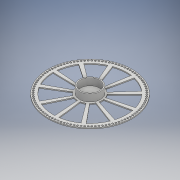
# Autodesk Inventor part: WheeledGrabber
Saved by Autodesk Inventor 2017 (Build 210142000, 142)
## iProperties
Created: 2017-01-07
Part Number: WheeledGrabber
Material: Generic
Document SubType Name: Modeling
Designer: kurti
Density: 1 g/cm^3
Appearance: Default
Author: kurti
Autodesk Inventor part; units mm, degrees
ref_plane "YZ Plane" through (0, 0, 0) normal (1, 0, 0) x (0, 1, 0)
ref_plane "XZ Plane" through (0, 0, 0) normal (0, 1, 0) x (-1, 0, 0)
ref_plane "XY Plane" through (0, 0, 0) normal (0, 0, 1) x (1, 0, 0)
sketch "Sketch1" plane through (0, 0, 0) normal (0, 0, 1) x (1, 0, 0)
  circle A0 centre (0, 0) radius 120
  line L0 (0, 0) -> (0, 115) construction
  circle A1 centre (0, 115) radius 2.5
  circle A2 centre (-7.2209, 114.7731) radius 2.5
  circle A3 centre (-14.4133, 114.0932) radius 2.5
  circle A4 centre (-21.5489, 112.963) radius 2.5
  circle A5 centre (-28.5993, 111.3871) radius 2.5
  circle A6 centre (-35.537, 109.3715) radius 2.5
  circle A7 centre (-42.3343, 106.9243) radius 2.5
  circle A8 centre (-48.9646, 104.0551) radius 2.5
  circle A9 centre (-55.4017, 100.7753) radius 2.5
  circle A10 centre (-61.6201, 97.0977) radius 2.5
  circle A11 centre (-67.5953, 93.037) radius 2.5
  circle A12 centre (-73.3038, 88.609) radius 2.5
  circle A13 centre (-78.7229, 83.8314) radius 2.5
  circle A14 centre (-83.8314, 78.7229) radius 2.5
  circle A15 centre (-88.609, 73.3038) radius 2.5
  circle A16 centre (-93.037, 67.5953) radius 2.5
  circle A17 centre (-97.0977, 61.6201) radius 2.5
  circle A18 centre (-100.7753, 55.4017) radius 2.5
  circle A19 centre (-104.0551, 48.9646) radius 2.5
  circle A20 centre (-106.9243, 42.3343) radius 2.5
  circle A21 centre (-109.3715, 35.537) radius 2.5
  circle A22 centre (-111.3871, 28.5993) radius 2.5
  circle A23 centre (-112.963, 21.5489) radius 2.5
  circle A24 centre (-114.0932, 14.4133) radius 2.5
  circle A25 centre (-114.7731, 7.2209) radius 2.5
  circle A26 centre (-115, 0) radius 2.5
  circle A27 centre (-114.7731, -7.2209) radius 2.5
  circle A28 centre (-114.0932, -14.4133) radius 2.5
  circle A29 centre (-112.963, -21.5489) radius 2.5
  circle A30 centre (-111.3871, -28.5993) radius 2.5
  circle A31 centre (-109.3715, -35.537) radius 2.5
  circle A32 centre (-106.9243, -42.3343) radius 2.5
  circle A33 centre (-104.0551, -48.9646) radius 2.5
  circle A34 centre (-100.7753, -55.4017) radius 2.5
  circle A35 centre (-97.0977, -61.6201) radius 2.5
  circle A36 centre (-93.037, -67.5953) radius 2.5
  circle A37 centre (-88.609, -73.3038) radius 2.5
  circle A38 centre (-83.8314, -78.7229) radius 2.5
  circle A39 centre (-78.7229, -83.8314) radius 2.5
  circle A40 centre (-73.3038, -88.609) radius 2.5
  circle A41 centre (-67.5953, -93.037) radius 2.5
  circle A42 centre (-61.6201, -97.0977) radius 2.5
  circle A43 centre (-55.4017, -100.7753) radius 2.5
  circle A44 centre (-48.9646, -104.0551) radius 2.5
  circle A45 centre (-42.3343, -106.9243) radius 2.5
  circle A46 centre (-35.537, -109.3715) radius 2.5
  circle A47 centre (-28.5993, -111.3871) radius 2.5
  circle A48 centre (-21.5489, -112.963) radius 2.5
  circle A49 centre (-14.4133, -114.0932) radius 2.5
  circle A50 centre (-7.2209, -114.7731) radius 2.5
  circle A51 centre (0, -115) radius 2.5
  circle A52 centre (7.2209, -114.7731) radius 2.5
  circle A53 centre (14.4133, -114.0932) radius 2.5
  circle A54 centre (21.5489, -112.963) radius 2.5
  circle A55 centre (28.5993, -111.3871) radius 2.5
  circle A56 centre (35.537, -109.3715) radius 2.5
  circle A57 centre (42.3343, -106.9243) radius 2.5
  circle A58 centre (48.9646, -104.0551) radius 2.5
  circle A59 centre (55.4017, -100.7753) radius 2.5
  circle A60 centre (61.6201, -97.0977) radius 2.5
  circle A61 centre (67.5953, -93.037) radius 2.5
  circle A62 centre (73.3038, -88.609) radius 2.5
  circle A63 centre (78.7229, -83.8314) radius 2.5
  circle A64 centre (83.8314, -78.7229) radius 2.5
  circle A65 centre (88.609, -73.3038) radius 2.5
  circle A66 centre (93.037, -67.5953) radius 2.5
  circle A67 centre (97.0977, -61.6201) radius 2.5
  circle A68 centre (100.7753, -55.4017) radius 2.5
  circle A69 centre (104.0551, -48.9646) radius 2.5
  circle A70 centre (106.9243, -42.3343) radius 2.5
  circle A71 centre (109.3715, -35.537) radius 2.5
  circle A72 centre (111.3871, -28.5993) radius 2.5
  circle A73 centre (112.963, -21.5489) radius 2.5
  circle A74 centre (114.0932, -14.4133) radius 2.5
  circle A75 centre (114.7731, -7.2209) radius 2.5
  circle A76 centre (115, 0) radius 2.5
  circle A77 centre (114.7731, 7.2209) radius 2.5
  circle A78 centre (114.0932, 14.4133) radius 2.5
  circle A79 centre (112.963, 21.5489) radius 2.5
  circle A80 centre (111.3871, 28.5993) radius 2.5
  circle A81 centre (109.3715, 35.537) radius 2.5
  circle A82 centre (106.9243, 42.3343) radius 2.5
  circle A83 centre (104.0551, 48.9646) radius 2.5
  circle A84 centre (100.7753, 55.4017) radius 2.5
  circle A85 centre (97.0977, 61.6201) radius 2.5
  circle A86 centre (93.037, 67.5953) radius 2.5
  circle A87 centre (88.609, 73.3038) radius 2.5
  circle A88 centre (83.8314, 78.7229) radius 2.5
  circle A89 centre (78.7229, 83.8314) radius 2.5
  circle A90 centre (73.3038, 88.609) radius 2.5
  circle A91 centre (67.5953, 93.037) radius 2.5
  circle A92 centre (61.6201, 97.0977) radius 2.5
  circle A93 centre (55.4017, 100.7753) radius 2.5
  circle A94 centre (48.9646, 104.0551) radius 2.5
  circle A95 centre (42.3343, 106.9243) radius 2.5
  circle A96 centre (35.537, 109.3715) radius 2.5
  circle A97 centre (28.5993, 111.3871) radius 2.5
  circle A98 centre (21.5489, 112.963) radius 2.5
  circle A99 centre (14.4133, 114.0932) radius 2.5
  circle A100 centre (7.2209, 114.7731) radius 2.5
  line L1 (0, 0) -> (90.9327, 52.5) construction
  line L2 (0, 0) -> (105, 0) construction
  line L3 (90.9327, 52.5) -> (8.6603, 5) construction
  line L4 (8.6603, 5) -> (75.8354, 72.1751)
  line L5 (8.6603, 5) -> (100.4232, 29.5878)
  line L6 (8.6603, 5) -> (103.6603, 5) construction
  arc A101 (100.4232, 29.5878) -> (75.8354, 72.1751) centre (-0.2751, -0.1588) ccw
  line L7 (4.4527, 9.0118) -> (24.6465, 101.8408)
  arc A102 (68.3555, 79.3072) -> (24.6465, 101.8408) centre (-0.2751, -0.1588) ccw
  line L8 (4.4527, 9.0118) -> (68.3555, 79.3072)
  line L9 (-1.2558, 10.1121) -> (-34.4549, 99.1223)
  arc A103 (14.498, 103.7967) -> (-34.4549, 99.1223) centre (-0.2751, -0.1588) ccw
  line L10 (-1.2558, 10.1121) -> (14.498, 103.7967)
  line L11 (-6.653, 7.9514) -> (-82.7044, 64.8828)
  arc A104 (-44.0497, 95.2811) -> (-82.7044, 64.8828) centre (-0.2751, -0.1588) ccw
  line L12 (-6.653, 7.9514) -> (-44.0497, 95.2811)
  line L13 (-10.0252, 3.2158) -> (-104.7831, 9.993)
  arc A105 (-88.6994, 56.464) -> (-104.7831, 9.993) centre (-0.2751, -0.1588) ccw
  line L14 (-10.0252, 3.2158) -> (-88.6994, 56.464)
  line L15 (-10.3018, -2.5913) -> (-93.6813, -48.1199)
  arc A106 (-105.2749, -0.3305) -> (-93.6813, -48.1199) centre (-0.2751, -0.1588) ccw
  line L16 (-10.3018, -2.5913) -> (-105.2749, -0.3305)
  line L17 (-7.395, -7.626) -> (-52.9237, -91.0055)
  arc A107 (-88.5137, -57.0704) -> (-52.9237, -91.0055) centre (-0.2751, -0.1588) ccw
  line L18 (-7.395, -7.626) -> (-88.5137, -57.0704)
  line L19 (-2.2277, -10.2899) -> (4.5496, -105.0479)
  arc A108 (-43.7374, -95.7414) -> (4.5496, -105.0479) centre (-0.2751, -0.1588) ccw
  line L20 (-2.2277, -10.2899) -> (-43.7374, -95.7414)
  line L21 (3.5596, -9.7373) -> (60.491, -85.7887)
  arc A109 (14.8379, -104.0655) -> (60.491, -85.7887) centre (-0.2751, -0.1588) ccw
  line L22 (3.5596, -9.7373) -> (14.8379, -104.0655)
  line L23 (8.1294, -6.1436) -> (97.1396, -39.3427)
  arc A110 (68.615, -79.4) -> (97.1396, -39.3427) centre (-0.2751, -0.1588) ccw
  line L24 (8.1294, -6.1436) -> (68.615, -79.4)
  line L25 (10.0309, -0.6497) -> (102.8598, 19.544)
  arc A111 (100.5199, -29.5759) -> (102.8598, 19.544) centre (-0.2751, -0.1588) ccw
  line L26 (10.0309, -0.6497) -> (100.5199, -29.5759)
  circle A112 centre (-0.2751, -0.1588) radius 35
  dimension "d0" = 240
  dimension "d1" = 115
  dimension "d2" = 5
  dimension "d5" = 360
  dimension "d13" = 105
  dimension "d14" = 30
  dimension "d15" = 95
  dimension "d16" = 95
  dimension "d17" = 15
  dimension "d18" = 95
  dimension "d19" = 15
  dimension "d20" = 105
  dimension "d23" = 360
  dimension "d25" = 70
  constraints: 113 centre point, 54 end point, 22 point on circle, 5 coincident, 2 equal length, 2 horizontal, 1 point on line, 1 vertical, 277 other
  measures "d0" diameter of A0
  measures "d1" distance of L0.start L0.end
  measures "d2" diameter of A1
  measures "d13" distance of L0.start L1.end
  measures "d14" angle of L2 L1
  measures "d15" distance of L1.end L3.end
  measures "d16" distance of L3.end L4.end
  measures "d17" angle of L3 L4
  measures "d18" distance of L3.end L5.end
  measures "d19" angle of L6 L5
  measures "d20" radius of A101
  measures "d25" diameter of A112
extrude "Extrusion1" add sketch "Sketch1" along normal blind 3 contours A0 | L5 A112 L25 L26 L23 L24 L21 L22 L19 L20 L17 L18 L15 L16 L13 L14 L11 L12 L9 L10 L7 L8 L4 | L4 A112 L5 | L8 L7 A112 | A112 L26 L25 | L10 L9 A112 | A112 L24 L23 | L12 L11 A112 | A112 L22 L21 | L14 L13 A112 | A112 L20 L19 | L16 L15 A112 | A112 L18 L17
sketch "Sketch2" plane through (0, 0, 3) normal (0, 0, 1) x (1, 0, 0)
  circle A0 centre (0, 0) radius 27
  circle A1 centre (0, 0) radius 30
  dimension "d9" = 54
  dimension "d10" = 60
  constraints: 2 centre point, 2 coincident
  measures "d9" diameter of A0
  measures "d10" diameter of A1
extrude "Extrusion2" add sketch "Sketch2" along normal blind 20
body "Solid1"
